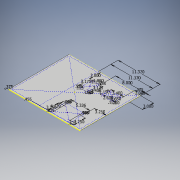
# Autodesk Inventor part: nmt_bottom
Saved by Autodesk Inventor 2017 (Build 210142000, 142)
## iProperties
Created: 2017-02-17
Part Number: nmt_bottom
Material: Generic
Document SubType Name: Modeling
Designer: Zara
Density: 1 g/cm^3
Appearance: Default
Author: Zara
Autodesk Inventor part; units mm, degrees
ref_plane "YZ Plane" through (0, 0, 0) normal (1, 0, 0) x (0, 1, 0)
ref_plane "XZ Plane" through (0, 0, 0) normal (0, 1, 0) x (-1, 0, 0)
ref_plane "XY Plane" through (0, 0, 0) normal (0, 0, 1) x (1, 0, 0)
sketch "Sketch1" plane through (0, 0, 0) normal (0, 1, 0) x (-1, 0, 0)
  line L0 (-245.999, 208.915) -> (245.999, 208.915)
  line L1 (245.999, 208.915) -> (245.999, -208.915)
  line L2 (245.999, -208.915) -> (-245.999, -208.915)
  line L3 (-245.999, -208.915) -> (-245.999, 208.915)
  line L4 (-245.999, 208.915) -> (245.999, -208.915) construction
  line L5 (245.999, 208.915) -> (-245.999, -208.915) construction
  point P0 (0, 0)
  dimension "d0" = 417.83
  dimension "d1" = 491.998
  constraints: 12 end point, 2 midpoint, 2 parallel, 1 horizontal, 1 perpendicular
  measures "d0" distance of L2.end L0.start
  measures "d1" distance of L1.end L2.end
extrude "Extrusion1" add sketch "Sketch1" along normal blind 1.778
sketch "wr" plane through (0, 1.778, 0) normal (0, 1, 0) x (1, 0, 0)
  line L0 (236.474, -199.39) -> (-236.474, -199.39) construction
  line L1 (-236.474, -199.39) -> (-236.474, 199.39) construction
  line L2 (-236.474, 199.39) -> (236.474, 199.39) construction
  line L3 (236.474, 199.39) -> (236.474, -199.39) construction
  line L4 (236.474, -199.39) -> (-236.474, 199.39) construction
  line L5 (-236.474, -199.39) -> (236.474, 199.39) construction
  line L6 (-245.999, -208.915) -> (245.999, -208.915) construction
  line L7 (245.999, -208.915) -> (245.999, 208.915) construction
  line L8 (163.449, -197.358) -> (28.1686, -197.358) construction
  line L9 (28.1686, -197.358) -> (28.1686, -92.2274) construction
  line L10 (28.1686, -92.2274) -> (163.449, -92.2274) construction
  line L11 (163.449, -92.2274) -> (163.449, -197.358) construction
  line L12 (163.449, -197.358) -> (28.1686, -92.2274) construction
  line L13 (28.1686, -197.358) -> (163.449, -92.2274) construction
  point P0 (0, 0)
  point P1 (95.8088, -144.7927)
  point P2 (95.8088, -144.7927)
  point P3 (150.749, -181.483)
  point P4 (40.8686, -181.483)
  point P5 (40.8686, -114.808)
  point P6 (150.749, -114.808)
  dimension "d4" = 9.525
  dimension "d5" = 9.525
  dimension "d6" = 105.1306
  dimension "d7" = 135.2804
  dimension "d9" = 11.557
  dimension "d10" = 82.55
  dimension "d23" = 15.875
  dimension "d24" = 15.875
  dimension "d25" = 12.7
  dimension "d26" = 12.7
  dimension "d27" = 82.55
  dimension "d28" = 82.55
  dimension "d29" = 12.7
  dimension "d30" = 12.7
  constraints: 24 end point, 5 midpoint, 4 parallel, 2 horizontal, 2 perpendicular
  measures "d4" distance between parallel lines of L6 L0
  measures "d5" distance between parallel lines of L7 L3
  measures "d6" distance of L8.end L9.end
  measures "d7" distance of L9.end L10.end
  measures "d9" distance between parallel lines of L6 L8
  measures "d10" distance between parallel lines of L7 L11
  measures "d23" distance from line of L8 point (150.749, -181.483)
  measures "d24" distance from line of L8 point (40.869, -181.483)
  measures "d25" distance from line of point (150.749, -181.483) L11
  measures "d26" distance from line of L9 point (40.869, -181.483)
  measures "d27" distance from line of point (150.749, -114.808) L8
  measures "d28" distance from line of L8 point (40.869, -114.808)
  measures "d29" distance from line of point (150.749, -114.808) L11
  measures "d30" distance from line of point (40.869, -114.808) L9
sketch "bbb" plane through (0, 1.778, 0) normal (0, 1, 0) x (1, 0, 0)
  line L0 (-11.811, 46.355) -> (-11.811, 132.715) construction
  line L1 (-11.811, 132.715) -> (42.799, 132.715) construction
  line L2 (42.799, 132.715) -> (42.799, 46.355) construction
  line L3 (42.799, 46.355) -> (-11.811, 46.355) construction
  line L4 (-11.811, 46.355) -> (42.799, 132.715) construction
  line L5 (-11.811, 132.715) -> (42.799, 46.355) construction
  line L6 (245.999, 208.915) -> (-245.999, 208.915) construction
  line L7 (245.999, -208.915) -> (245.999, 208.915) construction
  line L8 (-42.799, -208.915) -> (-42.799, 208.915) construction
  point P0 (0, 0)
  point P1 (15.494, 89.535)
  point P2 (39.624, 60.96)
  point P3 (-8.636, 60.96)
  point P4 (36.449, 127)
  point P5 (-5.461, 127)
  dimension "d11" = 54.61
  dimension "d12" = 86.36
  dimension "d13" = 14.605
  dimension "d14" = 14.605
  dimension "d15" = 3.175
  dimension "d16" = 3.175
  dimension "d17" = 80.645
  dimension "d18" = 6.35
  dimension "d19" = 80.645
  dimension "d20" = 48.26
  dimension "d82" = 203.2
  dimension "d83" = 76.2
  dimension "d84" = 288.798
  constraints: 14 end point, 2 midpoint, 2 parallel, 2 perpendicular, 1 point on line
  measures "d11" distance of L0.end L1.end
  measures "d12" distance of L1.end L2.end
  measures "d13" distance from line of point (39.624, 60.96) L3
  measures "d14" distance from line of point (-8.636, 60.96) L3
  measures "d15" distance from line of point (39.624, 60.96) L2
  measures "d16" distance from line of point (-8.636, 60.96) L0
  measures "d17" distance from line of point (36.449, 127) L3
  measures "d18" distance from line of point (36.449, 127) L2
  measures "d19" distance from line of point (-5.461, 127) L3
  measures "d20" distance from line of point (-5.461, 127) L2
  measures "d82" distance between parallel lines of L7 L2
  measures "d83" distance between parallel lines of L6 L1
  measures "d84" distance between parallel lines of L7 L8
sketch "Sketch5" plane through (0, 0, 0) normal (0, -1, 0) x (1, 0, 0)
  point P0 (0, 0)
  point P1 (36.449, -127)
  point P2 (-5.461, -127)
  point P3 (-8.636, -60.96)
  point P4 (39.624, -60.96)
sketch "bbb bob" plane through (0, 1.778, 0) normal (0, 1, 0) x (1, 0, 0)
  line L0 (245.999, -208.915) -> (-245.999, -208.915) projected
  line L1 (-42.799, -208.915) -> (-42.799, 208.1802) construction
  line L2 (245.999, -208.915) -> (245.999, 208.915) construction
  line L3 (195.199, 78.105) -> (108.839, 78.105) construction
  line L4 (108.839, 78.105) -> (108.839, 132.715) construction
  line L5 (108.839, 132.715) -> (195.199, 132.715) construction
  line L6 (195.199, 132.715) -> (195.199, 78.105) construction
  line L7 (195.199, 78.105) -> (108.839, 132.715) construction
  line L8 (108.839, 78.105) -> (195.199, 132.715) construction
  line L9 (245.999, 208.915) -> (-245.999, 208.915) construction
  point P0 (0, 0)
  point P1 (152.019, 105.41)
  point P2 (180.594, 84.455)
  point P3 (180.594, 126.365)
  point P4 (114.554, 84.455)
  point P5 (114.554, 126.365)
  dimension "d45" = 288.798
  dimension "d60" = 54.61
  dimension "d61" = 86.36
  dimension "d62" = 76.2
  dimension "d63" = 50.8
  dimension "d65" = 14.605
  dimension "d66" = 6.35
  dimension "d69" = 41.91
  dimension "d72" = 66.04
  constraints: 14 end point, 2 horizontal, 2 midpoint, 2 parallel, 2 vertical, 1 perpendicular, 1 point on line, 3 other
  measures "d45" distance between parallel lines of L2 L1
  measures "d60" distance of L3.end L4.end
  measures "d61" distance of L4.end L5.end
  measures "d62" distance between parallel lines of L9 L5
  measures "d63" distance between parallel lines of L6 L2
  measures "d65" distance from line of point (180.594, 84.455) L6
  measures "d66" distance from line of point (180.594, 84.455) L3
  measures "d69" distance of point (180.594, 84.455) point (180.594, 126.365)
  measures "d72" distance of point (180.594, 84.455) point (114.554, 84.455)
sketch "Sketch7" plane through (0, 0, 0) normal (0, -1, 0) x (1, 0, 0)
  point P0 (0, 0)
  point P1 (40.8686, 181.483)
  point P2 (40.8686, 114.808)
  point P3 (150.749, 181.483)
  point P4 (150.749, 114.808)
hole "wrlen holes" at (40.8686, 0, 114.808) at (40.8686, 0, 181.483) at (150.749, 0, 181.483) at (150.749, 0, 114.808) direction (0, 1, 0) diameter 3.4036 end through all countersink diameter 6.2992 countersink angle 90 clearance for "Countersunk Flat Head Screw ISO 2009/7046" size "M3" standard "ISO"
sketch "Sketch8" plane through (0, 0, 0) normal (0, -1, 0) x (1, 0, 0)
  point P0 (0, 0)
  point P1 (114.554, -126.365)
  point P2 (114.554, -84.455)
  point P3 (180.594, -126.365)
  point P4 (180.594, -84.455)
hole "bbb holes" at (-5.461, 0, -127) at (-8.636, 0, -60.96) at (39.624, 0, -60.96) at (36.449, 0, -127) direction (0, 1, 0) diameter 2.9 end through all countersink diameter 5.5 countersink angle 90 clearance for "Countersunk Flat Head Screw ISO 2009/7046" size "M2.5" standard "ISO"
hole "bbb bob holes" at (114.554, 0, -126.365) at (114.554, 0, -84.455) at (180.594, 0, -84.455) at (180.594, 0, -126.365) direction (0, 1, 0) diameter 2.9 end through all countersink diameter 5.5 countersink angle 90 clearance for "Countersunk Flat Head Screw ISO 2009/7046" size "M2.5" standard "ISO"
body "Solid1"
